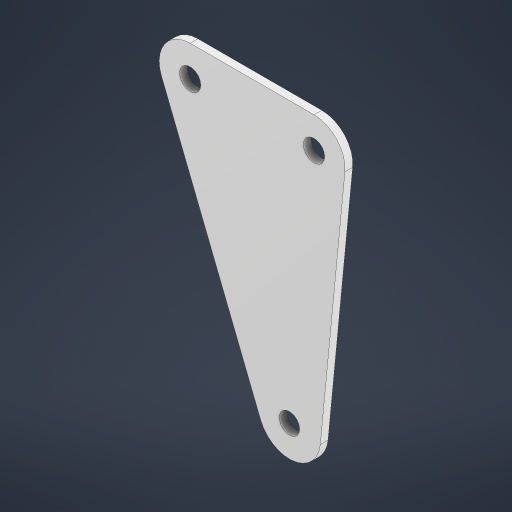
# Autodesk Inventor part: vertical_wing_gusset
Saved by Autodesk Inventor 2024 (Build 280153000, 153)
## iProperties
Created: 2024-01-17
Part Number: vertical_wing_gusset
Material: Acetal Resin, White
Document SubType Name: Modeling
Designer: avere
Density: 1.425 g/cm^3
Appearance: Smooth - White
Author: avere
Autodesk Inventor part; units mm, degrees
ref_plane "YZ Plane" through (0, 0, 0) normal (1, 0, 0) x (0, 1, 0)
ref_plane "XZ Plane" through (0, 0, 0) normal (0, 1, 0) x (-1, 0, 0)
ref_plane "XY Plane" through (0, 0, 0) normal (0, 0, 1) x (1, 0, 0)
sketch "main" plane through (0, 0, 0) normal (0, 0, 1) x (1, 0, 0)
  circle A0 centre (11.6396, 18.419) radius 2.1844
  circle A1 centre (-13.7604, 18.419) radius 2.1844
  arc A2 (-13.7604, 24.769) -> (-19.6572, 16.0633) centre (-13.7604, 18.419) ccw
  arc A3 (17.9587, 17.7933) -> (11.6396, 24.769) centre (11.6396, 18.419) ccw
  line L0 (-19.6572, 16.0633) -> (0.6972, -34.8883)
  line L1 (17.9587, 17.7933) -> (12.9132, -33.1583)
  line L2 (-13.7604, 24.769) -> (11.6396, 24.769)
  circle A4 centre (6.5941, -32.5326) radius 2.0955
  arc A5 (0.6972, -34.8883) -> (12.9132, -33.1583) centre (6.5941, -32.5326) ccw
  point P0 (1.7688, 7.28)
  dimension "d0" = 12.7
  dimension "d1" = 12.7
  dimension "d2" = 12.7
  dimension "d5" = 4.191
  measures "d0" diameter of A2
  measures "d1" diameter of A3
  measures "d2" diameter of A5
  measures "d5" diameter of A4
sketch "Sketch1" plane through (0, 0, 0) normal (0, 0, 1) x (1, 0, 0)
  circle A0 centre (25.4, 0) radius 2.1844
  circle A1 centre (0, 0) radius 2.1844
  arc A2 (0, 6.35) -> (-5.8969, -2.3557) centre (0, 0) ccw
  arc A3 (31.7191, -0.6258) -> (25.4, 6.35) centre (25.4, 0) ccw
  line L0 (-5.8969, -2.3557) -> (14.4576, -53.3073)
  line L1 (31.7191, -0.6258) -> (26.6735, -51.5774)
  line L2 (0, 6.35) -> (25.4, 6.35)
  circle A4 centre (20.3545, -50.9516) radius 2.0955
  arc A5 (14.4576, -53.3073) -> (26.6735, -51.5774) centre (20.3545, -50.9516) ccw
  constraints: 1 other
extrude "Extrusion1" add sketch "Sketch1" along normal blind 1.5875
body "Solid1"
